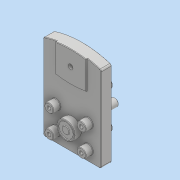
# Autodesk Inventor part: Giảm tốc DC 775
Saved by Autodesk Inventor 2018 (Build 220112000, 112)
## iProperties
Created: 2020-08-11
Part Number: Giảm tốc DC 775
Material: Generic
Document SubType Name: Modeling
Designer: ASUS
Density: 1 g/cm^3
Appearance: Default
Author: ASUS
Autodesk Inventor part; units mm, degrees
ref_plane "YZ Plane" through (0, 0, 0) normal (1, 0, 0) x (0, 1, 0)
ref_plane "XZ Plane" through (0, 0, 0) normal (0, 1, 0) x (-1, 0, 0)
ref_plane "XY Plane" through (0, 0, 0) normal (0, 0, 1) x (1, 0, 0)
sketch "Sketch1" plane through (0, 0, 0) normal (0, 1, 0) x (-1, 0, 0)
  line L0 (30.5, 45) -> (-30.5, 45)
  line L1 (-30.5, 45) -> (-30.5, -45)
  line L2 (-30.5, -45) -> (30.5, -45)
  line L3 (30.5, -45) -> (30.5, 45)
  line L4 (30.5, 45) -> (-30.5, -45) construction
  line L5 (-30.5, 45) -> (30.5, -45) construction
  arc A0 (30.5, 45) -> (-30.5, 45) centre (0, -46.0261) ccw
  point P0 (0, 0)
  dimension "d0" = 61
  dimension "d1" = 90
  dimension "d3" = 96
  constraints: 12 end point, 2 midpoint, 2 parallel, 2 point on circle, 1 centre point, 1 horizontal, 1 perpendicular
  measures "d0" distance of L2.end L1.end
  measures "d1" distance of L1.end L0.end
  measures "d3" radius of A0
extrude "Extrusion1" add sketch "Sketch1" along normal blind 11
sketch "Sketch2" plane through (0, 11, 0) normal (0, 1, 0) x (1, 0, 0)
  circle A0 centre (0, 21.5) radius 9.5
  line L0 (30.5, 45) -> (-30.5, 45) projected
  point P0 (0, 0)
  dimension "d6" = 19
  dimension "d9" = 23.5
  constraints: 1 centre point
  measures "d6" diameter of A0
  measures "d9" distance from line of L0 A0.centre
extrude "Extrusion2" add sketch "Sketch2" along normal blind 7
sketch "Sketch3" plane through (0, 11, 0) normal (0, 1, 0) x (1, 0, 0)
  line L0 (-19.5, -19) -> (19.5, 20) construction
  line L1 (19.5, -19) -> (-19.5, 20) construction
  line L2 (30.5, 45) -> (-30.5, 45) projected
  circle A0 centre (-19.5, -19) radius 4.75
  circle A1 centre (-19.5, 20) radius 4.75
  circle A2 centre (19.5, -19) radius 4.75
  circle A3 centre (19.5, 20) radius 4.75
  circle A4 centre (-19.5, -19) radius 1.5
  circle A5 centre (19.5, -19) radius 1.5
  circle A6 centre (19.5, 20) radius 1.5
  circle A7 centre (-19.5, 20) radius 1.5
  point P0 (0, 0)
  point P1 (0, 0.5)
  dimension "d10" = 39
  dimension "d11" = 39
  dimension "d13" = 9.5
  dimension "d14" = 9.5
  dimension "d15" = 9.5
  dimension "d16" = 9.5
  dimension "d17" = 3
  dimension "d18" = 3
  dimension "d19" = 3
  dimension "d20" = 3
  constraints: 8 centre point, 8 coincident, 4 end point, 2 midpoint
  measures "d10" distance of L1.end L0.end
  measures "d11" distance of L0.end L1.start
  measures "d13" diameter of A0
  measures "d14" diameter of A1
  measures "d15" diameter of A2
  measures "d16" diameter of A3
  measures "d17" diameter of A4
  measures "d18" diameter of A5
  measures "d19" diameter of A6
  measures "d20" diameter of A7
extrude "Extrusion3" add sketch "Sketch3" along normal blind 7.5
sketch "Sketch4" plane through (0, 0, 0) normal (0, -1, 0) x (1, 0, 0)
  circle A0 centre (0, -21.5) radius 9.5 projected
  circle A1 centre (0, -21.5) radius 9.5
  point P0 (0, 0)
  constraints: 1 centre point, 1 coincident
extrude "Extrusion4" add sketch "Sketch4" along normal blind 7
sketch "Sketch5" plane through (0, 0, 0) normal (0, -1, 0) x (1, 0, 0)
  circle A0 centre (0, -21.5) radius 9.5 projected
  line L0 (17, -9.5) -> (-17, -33.5) construction
  line L1 (-17, -9.5) -> (17, -33.5) construction
  circle A1 centre (17, -9.5) radius 4.75
  circle A2 centre (17, -33.5) radius 4.75
  circle A3 centre (-17, -9.5) radius 4.75
  circle A4 centre (-17, -33.5) radius 4.75
  circle A5 centre (17, -9.5) radius 1.5
  circle A6 centre (17, -33.5) radius 1.5
  circle A7 centre (-17, -9.5) radius 1.5
  circle A8 centre (-17, -33.5) radius 1.5
  point P0 (0, 0)
  dimension "d25" = 34
  dimension "d26" = 24
  dimension "d27" = 9.5
  dimension "d28" = 9.5
  dimension "d29" = 9.5
  dimension "d30" = 9.5
  dimension "d31" = 3
  dimension "d32" = 3
  dimension "d33" = 3
  dimension "d34" = 3
  constraints: 8 centre point, 7 coincident, 4 end point, 2 midpoint
  measures "d25" distance of L1.end L0.end
  measures "d26" distance of L0.end L1.start
  measures "d27" diameter of A1
  measures "d28" diameter of A2
  measures "d29" diameter of A3
  measures "d30" diameter of A4
  measures "d31" diameter of A5
  measures "d32" diameter of A6
  measures "d33" diameter of A7
  measures "d34" diameter of A8
extrude "Extrusion5" add sketch "Sketch5" along normal blind 7.5 contours A1 | A2 | A3 | A4
sketch "Sketch6" plane through (0, -7, -21.5) normal (0, -1, 0) x (1, 0, 0)
  circle A0 centre (0, 0) radius 7.5
  point P0 (0, 21.5)
  dimension "d37" = 15
  constraints: 1 centre point
  measures "d37" diameter of A0
extrude "Extrusion6" cut sketch "Sketch6" against normal blind 0.5
sketch "Sketch7" plane through (0, 18, -21.5) normal (0, 1, 0) x (1, 0, 0)
  circle A0 centre (0, 0) radius 7.5
  point P0 (0, -21.5)
  dimension "d40" = 15
  constraints: 1 centre point
  measures "d40" diameter of A0
extrude "Extrusion7" cut sketch "Sketch7" against normal blind 0.5
sketch "Sketch8" plane through (0, -7, -21.5) normal (0, -1, 0) x (1, 0, 0)
  circle A0 centre (0, 0) radius 4
  point P0 (0, 21.5)
  dimension "d43" = 8
  constraints: 1 centre point
  measures "d43" diameter of A0
extrude "Extrusion8" add sketch "Sketch8" against normal blind 52
fillet "Fillet1" radius 0.5 15 edges at (12.25, -7.5, -9.5) (15.5, -7.5, -9.5) (12.25, -7.5, -33.5) (15.5, -7.5, -33.5) (-21.75, -7.5, -33.5) (-18.5, -7.5, -33.5) (-21.75, -7.5, -9.5) (-18.5, -7.5, -9.5) (-4, -7, -21.5) (-9.5, -7, -21.5) (-7.5, -7, -21.5) (-21.75, 0, -9.5) (12.25, 0, -9.5) (12.25, 0, -33.5) (-21.75, 0, -33.5)
fillet "Fillet2" radius 0.5 15 edges at (-9.5, 18, -21.5) (-7.5, 18, -21.5) (14.75, 18.5, -20) (18, 18.5, -20) (-24.25, 18.5, -20) (-21, 18.5, -20) (-9.5, 11, -21.5) (-24.25, 11, -20) (14.75, 11, -20) (14.75, 18.5, 19) (18, 18.5, 19) (14.75, 11, 19) (-24.25, 18.5, 19) (-24.25, 11, 19) (-21, 18.5, 19)
chamfer "Chamfer1" distance 0.5 angle 45 1 edges at (-4, 45, -21.5)
sketch "Sketch9" plane through (0, 0, 0) normal (0, -1, 0) x (1, 0, 0)
  line L0 (16, 50) -> (16, 19)
  line L1 (-16, 19) -> (-16, 50)
  line L2 (-16, 50) -> (16, 19) construction
  line L3 (16, 50) -> (-16, 19) construction
  line L4 (30.5, -45) -> (-30.5, -45) projected
  arc A0 (30.5, 45) -> (-30.5, 45) centre (0, -46.0261) ccw projected
  arc A1 (16, 48.6312) -> (-16, 48.6312) centre (0, -46.0261) ccw
  arc A2 (-16, 19) -> (16, 19) centre (0, 113.6573) ccw
  point P0 (0, 0)
  point P1 (0, 34.5)
  dimension "d53" = 32
  dimension "d54" = 31
  dimension "d56" = 96
  constraints: 8 end point, 6 point on circle, 2 centre point, 2 midpoint, 2 point on line, 1 parallel
  measures "d53" distance of L0.end L1.start
  measures "d54" distance of L0.start L0.end
  measures "d56" radius of A2
extrude "Extrusion9" add sketch "Sketch9" along normal blind 1.6
fillet "Fillet4" radius 0.5 13 edges at (-30.5, 0, 0) (-30.5, 11, 0) (0, 0, -45) (0, 11, -45) (30.5, 0, 0) (23.3208, 0, 47.0982) (-23.3208, 0, 47.0982) (0, -1.6, 49.9739) (0, -1.6, 17.6573) (-16, -1.6, 33.8156) (16, -1.6, 33.8156) (0, 11, 49.9739) (30.5, 11, 0)
fillet "Fillet4" radius 2 4 edges at (30.5, 5.5, -45) (-30.5, 5.5, -45) (30.5, 5.5, 45) (-30.5, 5.5, 45)
sketch "Sketch10" plane through (0, -1.6, 0) normal (0, -1, 0) x (1, 0, 0)
  circle A0 centre (0, 33.8156) radius 2.5
  point P0 (0, 0)
  dimension "d62" = 5
  constraints: 1 centre point
  measures "d62" diameter of A0
extrude "Extrusion10" cut sketch "Sketch10" against normal blind 10
body "Solid1"
